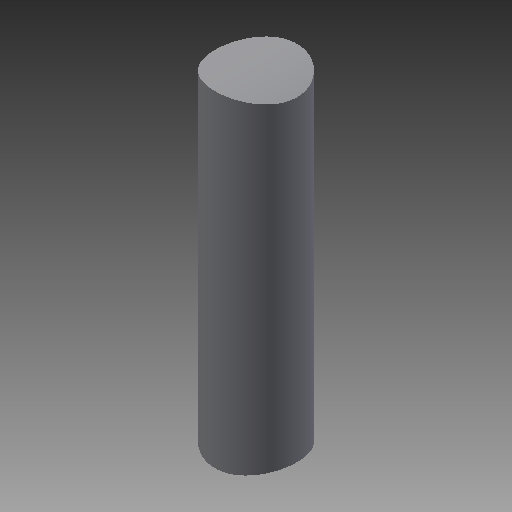
# Autodesk Inventor part: Piston Pin
Saved by Autodesk Inventor 2017 (Build 210142000, 142)
## iProperties
Created: 2012-08-14
Part Number: Piston Pin
Material: Generic
Document SubType Name: Modeling
Designer: John
Density: 1 g/cm^3
Appearance: Default
Author: John
Autodesk Inventor part; units mm, degrees
ref_plane "YZ Plane" through (0, 0, 0) normal (1, 0, 0) x (0, 1, 0)
ref_plane "XZ Plane" through (0, 0, 0) normal (0, 1, 0) x (-1, 0, 0)
ref_plane "XY Plane" through (0, 0, 0) normal (0, 0, 1) x (1, 0, 0)
sketch "Sketch1" plane through (0, 0, 0) normal (0, 1, 0) x (-1, 0, 0)
  circle A0 centre (0, 0) radius 1.7399
  dimension "d0" = 3.4798
  constraints: 1 centre point, 1 coincident
  measures "d0" diameter of A0
extrude "Extrusion1" add sketch "Sketch1" along normal mid plane 13.843
sketch "Sketch2" plane through (0, 0, 0) normal (0, 0, 1) x (1, 0, 0)
  line L0 (-1.7399, -6.9215) -> (1.7399, -6.9215) projected
  line L1 (1.7399, 6.9215) -> (-1.7399, 6.9215) projected
  line L2 (0, 6.9215) -> (0, -6.9215)
  circle A0 centre (0, 0) radius 6.9215
  circle A1 centre (0, 0) radius 7.1368
  constraints: 2 coincident, 2 end point, 2 midpoint, 1 vertical alignment, 5 other
extrude "Extrusion2" cut sketch "Sketch2" along normal through all both and the other way through all contours A1 L1 A0 L0 | L0 A1 | A0 L1 A1 L0 | A1 L1
body "Solid1"
